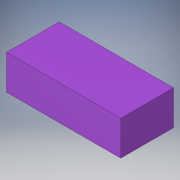
# Autodesk Inventor part: Q3_HC49UP
Saved by Autodesk Inventor 2017.3 (Build 213256000, 256)
## iProperties
Part Number: Q3_HC49UP
Material: Generisch
Document SubType Name: Modeling
Designer: Nils
Density: 1 g/cm^3
Appearance: HC49UP, Q3_HC49UP
Author: Nils
Autodesk Inventor part; units mm, degrees
ref_plane "YZ Plane" through (0, 0, 0) normal (1, 0, 0) x (0, 1, 0)
ref_plane "XZ Plane" through (0, 0, 0) normal (0, 1, 0) x (-1, 0, 0)
ref_plane "XY Plane" through (0, 0, 0) normal (0, 0, 1) x (1, 0, 0)
sketch "HC49UP, Q3_HC49UP_29" plane through (0, 0, 0) normal (0, 0, 1) x (1, 0, 0)
  line L0 (-6.604, 3.048) -> (6.604, 3.048)
  line L1 (6.604, 3.048) -> (6.604, -3.048)
  line L2 (6.604, -3.048) -> (-6.604, -3.048)
  line L3 (-6.604, -3.048) -> (-6.604, 3.048)
  constraints: 8 end point
extrude "Extrusion1" add sketch "HC49UP, Q3_HC49UP_29" along normal blind 4
